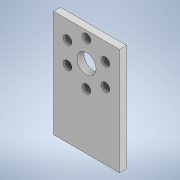
# Autodesk Inventor part: collection motor mount
Saved by Autodesk Inventor 2021 (Build 250183000, 183)
## iProperties
Created: 2021-01-07
Part Number: collection motor mount
Material: Generic
Document SubType Name: Modeling
Designer: User
Density: 1 g/cm^3
Appearance: Default
Author: User
Autodesk Inventor part; units mm, degrees
ref_plane "YZ Plane" through (0, 0, 0) normal (1, 0, 0) x (0, 1, 0)
ref_plane "XZ Plane" through (0, 0, 0) normal (0, 1, 0) x (-1, 0, 0)
ref_plane "XY Plane" through (0, 0, 0) normal (0, 0, 1) x (1, 0, 0)
sketch "Sketch1" plane through (0, 0, 0) normal (0, 0, 1) x (1, 0, 0)
  line L0 (0, 0) -> (24.13, 0)
  line L1 (24.13, 0) -> (24.13, 39.116)
  line L2 (24.13, 39.116) -> (0, 39.116)
  line L3 (0, 39.116) -> (0, 0)
  dimension "d0" = 39.116
  dimension "d1" = 24.13
  constraints: 8 end point, 2 parallel, 1 horizontal, 1 perpendicular
  measures "d0" distance of L0.end L1.end
  measures "d1" distance of L1.end L2.end
extrude "Extrusion1" add sketch "Sketch1" along normal blind 2.54
sketch "Sketch3" plane through (0, 0, 0) normal (0, -1, 0) x (1, 0, 0)
  circle A0 centre (3.9772, 1.2808) radius 0.9652
  circle A1 centre (20.3157, 1.2808) radius 0.9652
  point P0 (0, 0)
  dimension "d7" = 1.9304
  dimension "d8" = 1.9304
  constraints: 2 centre point
  measures "d7" diameter of A0
  measures "d8" diameter of A1
hole "Hole1" at (3.9772, 0, 1.2808) at (20.3157, 0, 1.2808) direction (0, 1, 0) diameter 1.6942 depth 5.7785 tip angle 118 thread size "2-56 UNC" class "2B" standard "ANSI Unified Screw Threads"
sketch "Sketch5" plane through (0, 0, 2.54) normal (0, 0, 1) x (1, 0, 0)
  circle A0 centre (12.065, 28.5714) radius 3.4925
  circle A1 centre (12.065, 28.5714) radius 8.001
  circle A2 centre (18.9941, 32.5719) radius 1.5875
  circle A3 centre (12.065, 36.5724) radius 1.5875
  circle A4 centre (12.065, 28.5714) radius 8.001
  circle A5 centre (5.1359, 32.5719) radius 1.5875
  circle A6 centre (12.065, 28.5714) radius 8.001
  circle A7 centre (5.1359, 24.5709) radius 1.5875
  circle A8 centre (12.065, 28.5714) radius 8.001
  circle A9 centre (12.065, 20.5704) radius 1.5875
  circle A10 centre (12.065, 28.5714) radius 8.001
  circle A11 centre (18.9941, 24.5709) radius 1.5875
  circle A12 centre (12.065, 28.5714) radius 8.001
  line L0 (24.13, 0) -> (24.13, 39.116) projected
  line L1 (24.13, 39.116) -> (0, 39.116) projected
  line L2 (0, 0) -> (24.13, 0) projected
  line L3 (12.065, 39.116) -> (12.065, 28.5714)
  dimension "d32" = 16.002
  dimension "d31" = 6.985
  dimension "d33" = 3.175
  dimension "d34" = 360
  dimension "d35" = 24.13
  constraints: 7 centre point, 2 coincident, 2 end point, 2 vertical alignment, 1 midpoint, 1 vertical, 41 other
  measures "d31" diameter of A0
  measures "d33" diameter of A2
  measures "d35" distance of L0.end L1.end
extrude "Extrusion4" cut sketch "Sketch5" against normal through all contours A0 | A3 A1 L3 | L3 A1 A3 | A3 L3 A1 | A1 L3 A3 | A5 A1 | A1 A5 | A2 A1 | A1 A2 | A7 A1 | A1 A7 | A11 A1 | A1 A11 | A9 A1 | A1 A9
body "Solid1"
